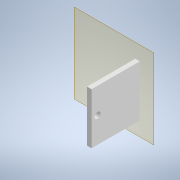
# Autodesk Inventor part: sideSupportFor12inchBase
Saved by Autodesk Inventor 2021 (Build 250183000, 183)
## iProperties
Created: 2020-07-01
Part Number: sideSupportFor12inchBase
Material: Generic
Document SubType Name: Modeling
Designer: robst
Density: 1 g/cm^3
Appearance: Default
Author: robst
Autodesk Inventor part; units mm, degrees
ref_plane "YZ Plane" through (0, 0, 0) normal (1, 0, 0) x (0, 1, 0)
ref_plane "XZ Plane" through (0, 0, 0) normal (0, 1, 0) x (-1, 0, 0)
ref_plane "XY Plane" through (0, 0, 0) normal (0, 0, 1) x (1, 0, 0)
ref_plane "Work Plane1" through (0, 0, 0) normal (0, 0, 1) x (1, 0, 0)
sketch "Sketch1" plane through (0, 0, 0) normal (0, 0, 1) x (1, 0, 0)
  circle A0 centre (0, 0) radius 152.4 projected
  line L0 (0.4005, -152.3995) -> (0.4005, 152.3995) construction
  line L1 (152.4, 0) -> (-152.4, 0) construction
  line L2 (107.95, 0) -> (107.95, -107.5758)
  line L3 (107.95, -107.5758) -> (88.9, -107.5758)
  line L4 (88.9, -107.5758) -> (88.9, 0)
  line L5 (107.95, 0) -> (107.95, 107.5758)
  line L6 (107.95, 107.5758) -> (88.9, 107.5758)
  line L7 (88.9, 107.5758) -> (88.9, 0)
  dimension "d0" = 19.05
  dimension "d2" = 88.9
  constraints: 16 end point, 5 point on circle, 2 horizontal, 2 perpendicular, 2 point on line, 2 symmetric about line, 1 vertical
  measures "d0" distance of L2.end L3.end
  measures "d2" distance from line of L4 point (0, 0)
extrude "Extrusion1" add sketch "Sketch1" along normal blind 203.2 contours L5 L2 L3 L4 L7 L6
sketch "Sketch2" plane through (107.95, -107.5758, 0) normal (1, 0, 0) x (0, 0, -1)
  line L0 (-203.2, 0) -> (-203.2, 215.1516) construction
  line L1 (-203.2, 107.5758) -> (0, 107.5758) construction
  circle A0 centre (-177.8, 107.5758) radius 12.7
  dimension "d5" = 25.4
  dimension "d6" = 25.4
  constraints: 2 end point, 1 centre point, 1 horizontal, 1 midpoint, 1 point on line
  measures "d5" diameter of A0
  measures "d6" distance from line of A0.centre L0
extrude "Extrusion2" cut sketch "Sketch2" against normal through all
body "Solid1"
